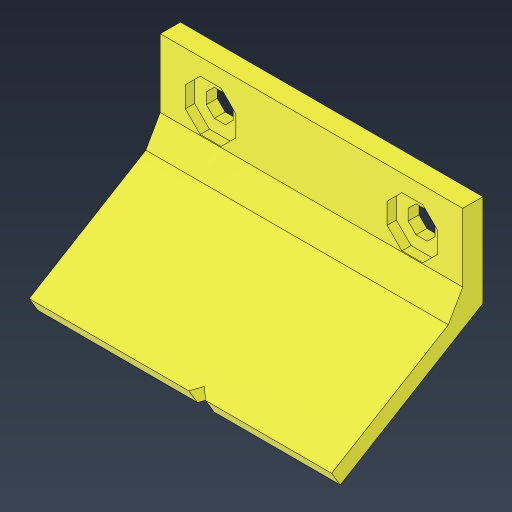
# Autodesk Inventor part: Dribblerdaempfer Flex
Saved by Autodesk Inventor 2023.1 (Build 271208000, 208)
## iProperties
Part Number: Dribblerdaempfer Flex
Material: Gummi, Silikon
Document SubType Name: Modeling
Designer: rYan
Density: 1.25 g/cm^3
Appearance: Glatt - Gelb
Mass: 2.53944 g
Surface Area: 25.4256 cm^2
Volume: 2.03155 cm^3
Author: rYan
Autodesk Inventor part; units mm, degrees
ref_plane "YZ Plane" through (0, 0, 0) normal (1, 0, 0) x (0, 1, 0)
ref_plane "XZ Plane" through (0, 0, 0) normal (0, 1, 0) x (-1, 0, 0)
ref_plane "XY Plane" through (0, 0, 0) normal (0, 0, 1) x (1, 0, 0)
sketch "Skizze1" plane through (0, 0, 0) normal (1, 0, 0) x (0, 1, 0)
  line L0 (0, -6) -> (0, 5)
  line L1 (0, 5) -> (-2.4, 5)
  line L2 (-2.4, 5) -> (-2.4, -5.1102)
  line L3 (-2.4, -5.1102) -> (-18, -14.5)
  line L4 (-18, -14.5) -> (-16.9686, -16.2135)
  line L5 (-16.9686, -16.2135) -> (0, -6)
  point P0 (0, 0)
  point P1 (0, -0.5)
  dimension "d0" = 5
  dimension "d1" = 2.4
  dimension "d3" = 14
  dimension "d4" = 18
  dimension "d12" = 2
  dimension "d15" = 6
  constraints: 12 end point, 4 perpendicular, 1 midpoint, 1 point on line, 1 vertical
  measures "d0" distance from line of L1 point (0, 0)
  measures "d1" distance of L0.end L1.end
  measures "d3" vertical distance of L3.end point (0, -0.5)
  measures "d4" horizontal distance of L3.end point (0, 0)
  measures "d12" distance between parallel lines of L5 L3
  measures "d15" distance of point (0, 0) L0.start
extrude "Extrusion1" add sketch "Skizze1" along normal mid plane 36
sketch "Skizze2" plane through (-18, -2.4, -5.1102) normal (0, -1, 0) x (1, 0, 0)
  line L0 (18, 14.3529) -> (18, -15.346) construction
  line L1 (31.6, 4.4475) -> (30.6627, 3.5102)
  line L2 (30.6627, 3.5102) -> (29.3373, 3.5102)
  line L3 (29.3373, 3.5102) -> (28.4, 4.4475)
  line L4 (28.4, 4.4475) -> (28.4, 5.773)
  line L5 (28.4, 5.773) -> (29.3373, 6.7102)
  line L6 (29.3373, 6.7102) -> (30.6627, 6.7102)
  line L7 (30.6627, 6.7102) -> (31.6, 5.773)
  line L8 (31.6, 5.773) -> (31.6, 4.4475)
  line L9 (7.6, 4.4475) -> (6.6627, 3.5102)
  line L10 (6.6627, 3.5102) -> (5.3373, 3.5102)
  line L11 (5.3373, 3.5102) -> (4.4, 4.4475)
  line L12 (4.4, 4.4475) -> (4.4, 5.773)
  line L13 (4.4, 5.773) -> (5.3373, 6.7102)
  line L14 (5.3373, 6.7102) -> (6.6627, 6.7102)
  line L15 (6.6627, 6.7102) -> (7.6, 5.773)
  line L16 (7.6, 5.773) -> (7.6, 4.4475)
  line L17 (-7.2, 5.1102) -> (43.2, 5.1102) construction
  point P0 (18, 5.1102)
  point P1 (30, 5.1102)
  point P2 (6, 5.1102)
  dimension "d8" = 3.2
  dimension "d9" = 24
  constraints: 32 end point, 1 collinear, 1 horizontal, 1 point on line, 1 symmetric about line, 34 other
  measures "d8" distance between parallel lines of L2 L6
  measures "d9" distance of point (6, 5.11) point (30, 5.11)
extrude "Extrusion2" cut sketch "Skizze2" against normal through all
chamfer "Fase1" distance 2 angle 45 1 edges at (0, -2.4, -5.1102)
sketch "Skizze3" plane through (-18, -2.4, 5) normal (0, -1, 0) x (1, 0, 0)
  line L0 (36, -8.1102) -> (0, -8.1102) projected
  line L1 (36, 0) -> (36, -8.1102) projected
  line L2 (0, 0) -> (36, 0) projected
  line L3 (0, -8.1102) -> (0, 0) projected
  line L4 (29.3373, -3.4) -> (30.6627, -3.4) projected
  line L5 (30.6627, -3.4) -> (31.6, -4.3373) projected
  line L6 (31.6, -4.3373) -> (31.6, -5.6627) projected
  line L7 (31.6, -5.6627) -> (30.6627, -6.6) projected
  line L8 (30.6627, -6.6) -> (29.3373, -6.6) projected
  line L9 (29.3373, -6.6) -> (28.4, -5.6627) projected
  line L10 (28.4, -5.6627) -> (28.4, -4.3373) projected
  line L11 (28.4, -4.3373) -> (29.3373, -3.4) projected
  line L12 (5.3373, -3.4) -> (6.6627, -3.4) projected
  line L13 (6.6627, -3.4) -> (7.6, -4.3373) projected
  line L14 (7.6, -4.3373) -> (7.6, -5.6627) projected
  line L15 (7.6, -5.6627) -> (6.6627, -6.6) projected
  line L16 (6.6627, -6.6) -> (5.3373, -6.6) projected
  line L17 (5.3373, -6.6) -> (4.4, -5.6627) projected
  line L18 (4.4, -5.6627) -> (4.4, -4.3373) projected
  line L19 (4.4, -4.3373) -> (5.3373, -3.4) projected
  line L20 (31.2426, -2) -> (28.7574, -2)
  line L21 (28.7574, -2) -> (27, -3.7574)
  line L22 (27, -3.7574) -> (27, -6.2426)
  line L23 (27, -6.2426) -> (28.7574, -8)
  line L24 (28.7574, -8) -> (31.2426, -8)
  line L25 (31.2426, -8) -> (33, -6.2426)
  line L26 (33, -6.2426) -> (33, -3.7574)
  line L27 (33, -3.7574) -> (31.2426, -2)
  point P0 (18, -5)
  point P1 (28.2105, -7.4531)
  point P2 (31.7895, -7.4531)
  dimension "d19" = 6
  constraints: 16 end point, 7 other
  measures "d19" distance between parallel lines of L26 L22
extrude "Extrusion3" cut sketch "Skizze3" along normal mid plane 2.2 contours L27 L26 L25 L24 L23 L22 L21 L20
mirror "Spiegeln1" about plane through (0, 0, 0) normal (1, 0, 0) of "Extrusion3"
sketch "Skizze4" plane through (-18, -18, -14.5) normal (0, -0.5156973, 0.8567708) x (1, 0, 0)
  line L0 (0, 16.2079) -> (36, 16.2079) projected
  line L1 (0, 0) -> (0, 16.2079) projected
  line L2 (0, 0) -> (36, 0) projected
  line L3 (36, 16.2079) -> (36, 0) projected
  line L4 (18, 32.4901) -> (18, -6.446) construction
  line L5 (19, 0) -> (20, 1)
  line L6 (20, 1) -> (21, 0)
  line L7 (20, 1) -> (20, 0) construction
  point P0 (18, 22.8995)
  dimension "d22" = 1
  dimension "d23" = 1
  constraints: 6 end point, 3 point on line, 2 perpendicular, 1 other
  measures "d22" distance of L5.end L7.end
  measures "d23" distance from line of L4 L5.start
extrude "Extrusion4" cut sketch "Skizze4" against normal through all contours L5 L6 L2
mirror "Spiegeln2" [suppressed]
